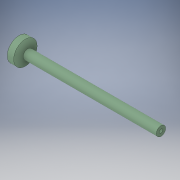
# Autodesk Inventor part: Rubber pipe
Saved by Autodesk Inventor 2019 (Build 230136000, 136)
## iProperties
Created: 2019-06-13
Part Number: Rubber pipe
Material: Generic
Document SubType Name: Sheet Metal
Designer: Satwik Pandey
Density: 1 g/cm^3
Sheet Metal Rule: Default_mm
Appearance: Rubber - Green
Author: Satwik Pandey
Autodesk Inventor part; units mm, degrees
ref_plane "YZ Plane" through (0, 0, 0) normal (1, 0, 0) x (0, 1, 0)
ref_plane "XZ Plane" through (0, 0, 0) normal (0, 1, 0) x (-1, 0, 0)
ref_plane "XY Plane" through (0, 0, 0) normal (0, 0, 1) x (1, 0, 0)
sketch "Sketch2" plane through (0, 0, 0) normal (0, 1, 0) x (-1, 0, 0)
  line L0 (-15, -3) -> (-165, -3)
  line L1 (-15, -8) -> (-165, -8)
  line L2 (146.5532, 0) -> (-237.9141, 0) projected
  line L3 (59.0935, -15) -> (59.0935, -20)
  line L4 (59.0935, -15) -> (48.2521, -15)
  line L5 (59.0935, -20) -> (48.2521, -20)
  arc A0 (44.0935, -3) -> (48.2521, -15) centre (91.6293, 6.7531) ccw
  arc A1 (44.0935, -8) -> (48.2521, -20) centre (72.6082, -4.8387) ccw
  line L6 (-165, -8) -> (-182.9902, -8)
  line L7 (-182.9902, -3) -> (-165, -3)
  line L8 (-182.9902, -8) -> (-182.9902, -3)
  line L9 (-15, -3) -> (5.213, -3)
  line L10 (-15, -8) -> (5.213, -8)
  line L11 (44.0935, -3) -> (5.213, -3)
  line L12 (5.213, -8) -> (44.0935, -8)
  point P0 (0, 0)
  point P1 (-13.1291, -22.6955)
  point P2 (-13.1263, -14.83)
  constraints: 24 end point, 4 parallel, 4 point on circle, 2 centre point, 2 horizontal, 1 collinear, 1 perpendicular
revolve "Revolution2" add sketch "Sketch2" angle 360 about axis through (-10, 0, 0) along (1, 0, 0)
equation "\"BendRadius\" = Thickness"
equation "\"BendReliefWidth\" = Thickness"
equation "\"BendReliefDepth\" = 0.5 * Thickness"
equation "\"CornerReliefSize\" = 4 * Thickness"
equation "\"MinimumRemnant\" = 2 * Thickness"
equation "\"TransitionRadius\" = BendRadius"
equation "\"JacobiRadiusSize\" = BendRadius"
equation "\"GapSize\" = Thickness"
equation "\"Thickness\" = 0.5"
body "Solid2"
